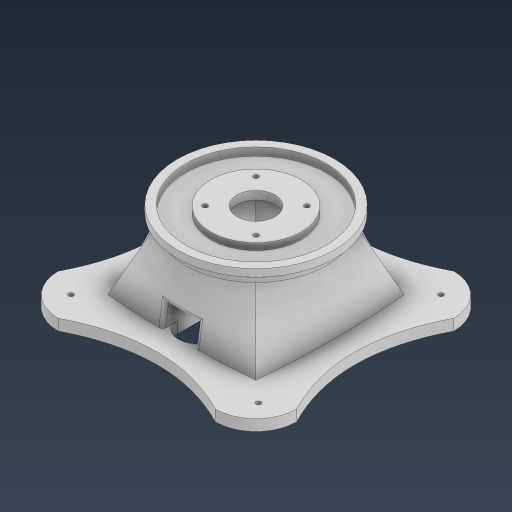
# Autodesk Inventor part: base_support
Saved by Autodesk Inventor 2024 (Build 280153000, 153)
## iProperties
Created: 2025-01-17
Part Number: base_support
Material: Generic
Document SubType Name: Modeling
Designer: Piter
Density: 1 g/cm^3
Appearance: Default
Author: Piter
Autodesk Inventor part; units mm, degrees
ref_plane "YZ Plane" through (0, 0, 0) normal (1, 0, 0) x (0, 1, 0)
sketch "Sketch1" plane through (0, 0, 0) normal (0, 1, 0) x (-1, 0, 0)
  circle A0 centre (0, 0) radius 27.35
  dimension "d0" = 54.7
  constraints: 1 centre point, 1 coincident
  measures "d0" diameter of A0
extrude "Extrusion1" add sketch "Sketch1" along normal blind 5
sketch "Sketch2" plane through (0, 0, 0) normal (0, -1, 0) x (1, 0, 0)
  circle A0 centre (0, 0) radius 47.5
  circle A1 centre (0, 0) radius 42.6
  circle A2 centre (0, 0) radius 27.35 projected
  dimension "d3" = 95
  dimension "d4" = 85.2
  constraints: 2 centre point, 2 coincident
  measures "d3" diameter of A0
  measures "d4" diameter of A1
extrude "Extrusion2" add sketch "Sketch2" along normal blind 5 and the other way blind 1 contours A1
extrude "Extrusion3" add sketch "Sketch2" along normal blind 2 and the other way blind 5.75 contours A0
chamfer "Chamfer1" distance 4.5 distance2 3.25 1 edges at (-47.5, -2, 0) measured on face at (-2.3305, -2, 44.0051)
ref_plane "Work Plane1" through (0, -48.5, 0) normal (0, -1, 0) x (1, 0, 0)
sketch "Sketch3" plane through (0, -48.5, 0) normal (0, -1, 0) x (1, 0, 0)
  line L0 (-47.5, 47.5) -> (47.5, 47.5)
  line L1 (47.5, 47.5) -> (47.5, -47.5)
  line L2 (47.5, -47.5) -> (-47.5, -47.5)
  line L3 (-47.5, -47.5) -> (-47.5, 47.5)
  line L4 (-47.5, 47.5) -> (47.5, -47.5) construction
  line L5 (47.5, 47.5) -> (-47.5, -47.5) construction
  line L6 (-22.5, 22.5) -> (22.5, 22.5)
  line L7 (22.5, 22.5) -> (22.5, -22.5)
  line L8 (22.5, -22.5) -> (-22.5, -22.5)
  line L9 (-22.5, -22.5) -> (-22.5, 22.5)
  circle A0 centre (0, 0) radius 27.35 projected
  line L10 (-22.5, 22.5) -> (22.5, -22.5) construction
  line L11 (22.5, 22.5) -> (-22.5, -22.5) construction
  dimension "d15" = 95
  dimension "d16" = 95
  dimension "d17" = 45
  dimension "d18" = 45
  constraints: 24 end point, 4 midpoint, 4 parallel, 2 horizontal, 2 perpendicular
  measures "d15" distance of L1.end L2.end
  measures "d16" distance of L0.end L1.end
  measures "d17" distance of L7.end L8.end
  measures "d18" distance of L6.end L7.end
sketch "Sketch4" plane through (0, -5, 0) normal (0, -1, 0) x (1, 0, 0)
  circle A0 centre (0, 0) radius 42.6 projected
  circle A1 centre (0, 0) radius 27.35 projected
sketch "Sketch5" plane through (0, -48.5, 0) normal (0, -1, 0) x (1, 0, 0)
  line L0 (-47.5, 47.5) -> (47.5, 47.5)
  line L1 (47.5, 47.5) -> (47.5, -47.5)
  line L2 (47.5, -47.5) -> (-47.5, -47.5)
  line L3 (-47.5, -47.5) -> (-47.5, 47.5)
  line L4 (-47.5, 47.5) -> (47.5, -47.5) construction
  line L5 (47.5, 47.5) -> (-47.5, -47.5) construction
  point P0 (0, 0)
  dimension "d21" = 95
  dimension "d22" = 95
  constraints: 12 end point, 2 midpoint, 2 parallel, 1 horizontal, 1 perpendicular
  measures "d21" distance of L1.end L2.end
  measures "d22" distance of L0.end L1.end
loft "Loft1" add profiles "Sketch5" section 2 edges at (-42.6, -5, 0)
extrude "Extrusion5" cut sketch "Sketch3" against normal blind 48.5 contours L6 A0 L9 | L6 A0 L7 L8 L9 | L6 L7 A0 | A0 L8 L9 | L7 L8 A0
ref_plane "Work Plane2" through (0, 2.25, 0) normal (0, 1, 0) x (1, 0, 0)
sketch "Sketch6" plane through (0, -5, 0) normal (0, 1, 0) x (1, 0, 0)
  line L0 (-15.549, 22.5) -> (15.549, 22.5) projected
  arc A0 (15.549, 22.5) -> (-15.549, 22.5) centre (0, 0) ccw projected
  line L1 (-22.5, -15.549) -> (-22.5, 15.549) projected
  arc A1 (-22.5, 15.549) -> (-22.5, -15.549) centre (0, 0) ccw projected
  line L2 (22.5, 15.549) -> (22.5, -15.549) projected
  arc A2 (22.5, -15.549) -> (22.5, 15.549) centre (0, 0) ccw projected
  line L3 (15.549, -22.5) -> (-15.549, -22.5) projected
  arc A3 (-15.549, -22.5) -> (15.549, -22.5) centre (0, 0) ccw projected
extrude "Extrusion6" add sketch "Sketch6" along normal blind 5
sketch "Sketch7" plane through (-47.5, -48.5, 47.5) normal (0, -1, 0) x (1, 0, 0)
  line L0 (0, 0) -> (95, 0) projected
  line L1 (95, 0) -> (77.6227, -17.3773) projected
  circle A0 centre (95, 0) radius 24.5751
  line L2 (95, -95) -> (0, -95) projected
  circle A1 centre (95, -95) radius 24.5751
  circle A2 centre (47.5, -47.5) radius 42.6 projected
  line L3 (0, -95) -> (17.3773, -77.6227) projected
  circle A3 centre (0, -95) radius 24.5751
  line L4 (0, 0) -> (17.3773, -17.3773) projected
  circle A4 centre (0, 0) radius 24.5751
  line L5 (95, 24.5751) -> (47.5, 0) construction
  line L6 (47.5, 0) -> (0, 24.5751) construction
  spline S0 degree 2 poles (95, 24.5751) (47.5, 0) (0, 24.5751) knots 1 1 1 2 2 2
  circle A5 centre (47.5, -47.5) radius 47.5 projected
  line L7 (-24.5751, 0) -> (0, -47.5) construction
  line L8 (0, -47.5) -> (-24.5751, -95) construction
  spline S1 degree 2 poles (-24.5751, 0) (0, -47.5) (-24.5751, -95) knots 1 1 1 2 2 2
  line L9 (0, -119.5751) -> (47.5, -95) construction
  line L10 (47.5, -95) -> (95, -119.5751) construction
  spline S2 degree 2 poles (0, -119.5751) (47.5, -95) (95, -119.5751) knots 1 1 1 2 2 2
  line L11 (119.5751, 0) -> (95, -47.5) construction
  line L12 (95, -47.5) -> (119.5751, -95) construction
  spline S3 degree 2 poles (119.5751, 0) (95, -47.5) (119.5751, -95) knots 1 1 1 2 2 2
  circle A6 centre (-8.3793, 8.3793) radius 1.5
  circle A7 centre (-8.3793, -103.3793) radius 1.5
  circle A8 centre (103.3793, -103.3793) radius 1.5
  circle A9 centre (104.8793, 8.3793) radius 1.5
  dimension "d47" = 3
  dimension "d48" = 3
  dimension "d49" = 3
  dimension "d50" = 3
  constraints: 14 point on circle, 8 centre point, 2 midpoint, 2 point on line, 1 coincident, 1 tangent, 12 other
  measures "d47" diameter of A6
  measures "d48" diameter of A7
  measures "d49" diameter of A8
  measures "d50" diameter of A9
extrude "Extrusion7" add sketch "Sketch7" against normal blind 7 contours L4 A5 A4 S1 S0 L0 | L0 A4 A5 L4 | A4 S0 A0 L0 | L0 A5 A4 | A5 A4 L4 | L4 A4 A5 | L0 A0 A5 | A5 A0 A2 A4 | A2 A3 A5 A4 | A5 A3 S1 A4 | A0 S0 S3 A5 L1 L0 | L0 L1 A5 A0 | A5 L1 A0 | L1 A5 A0 | A0 A5 A1 A2 | A3 A5 L3 | A2 A1 A5 A3 | L3 A5 A3 | A5 L3 L2 A3 S2 S1 | A0 S3 A1 A5 | A1 A5 | A5 A3 L2 L3 | A5 L2 A3 | A1 S3 S2 A5 | A1 L2 A5 | L2 A1 S2 A3
sketch "Sketch8" plane through (0, 5, 0) normal (0, 1, 0) x (1, 0, 0)
  circle A0 centre (0, 0) radius 11.5
  circle A1 centre (0, 0) radius 21.75
  line L0 (15.3796, -15.3796) -> (-15.3796, -15.3796)
  line L1 (-15.3796, -15.3796) -> (-15.3796, 15.3796)
  line L2 (-15.3796, 15.3796) -> (15.3796, 15.3796)
  line L3 (15.3796, 15.3796) -> (15.3796, -15.3796)
  line L4 (15.3796, -15.3796) -> (-15.3796, 15.3796) construction
  line L5 (-15.3796, -15.3796) -> (15.3796, 15.3796) construction
  circle A2 centre (-15.3796, 15.3796) radius 1.55
  circle A3 centre (15.3796, 15.3796) radius 1.55
  circle A4 centre (15.3796, -15.3796) radius 1.55
  circle A5 centre (-15.3796, -15.3796) radius 1.55
  dimension "d37" = 43.5
  dimension "d36" = 23
  dimension "d38" = 3.1
  dimension "d39" = 3.1
  dimension "d40" = 3.1
  dimension "d41" = 3.1
  constraints: 12 end point, 6 coincident, 5 centre point, 2 midpoint, 2 parallel, 2 perpendicular, 1 horizontal, 3 other
  measures "d36" diameter of A0
  measures "d38" diameter of A2
  measures "d39" diameter of A3
  measures "d40" diameter of A4
  measures "d41" diameter of A5
extrude "Extrusion8" cut sketch "Sketch8" against normal blind 10 contours A0 | A3 L3 A1 | A1 A3 | A4 A1 | A1 L3 A4 | L2 A3 A1 | L3 A3 L2 | A1 A4 L0 | L0 A4 L3 | A2 L2 A1 | A1 A2 | A2 L1 L2 | A5 A1 | A1 L0 A5 | L0 L1 A5 | L1 A2 A1 | A1 A5 L1
move faces "Move1" translate (0, 0.3, 0) faces at (-34.9452, -48.5, -0.9897)
sketch "Sketch9" plane through (22.5, 0, 22.5) normal (0, 0, -1) x (-1, 0, 0)
  point P0 (22.5, 0)
sketch "Sketch10" plane through (22.5, 0, 22.5) normal (0, 0, -1) x (-1, 0, 0)
  line L0 (0, -48.2) -> (0, 0) projected
  line L1 (0, -48.2) -> (45, -48.2)
  line L2 (22.5, -48.2) -> (22.5, -28.2)
  line L3 (12.5, -28.2) -> (32.5, -28.2)
  line L4 (32.5, -28.2) -> (32.5, -48.2)
  line L5 (32.5, -48.2) -> (12.5, -48.2)
  line L6 (12.5, -48.2) -> (12.5, -28.2)
  line L7 (12.5, -28.2) -> (32.5, -48.2) construction
  line L8 (32.5, -28.2) -> (12.5, -48.2) construction
  point P0 (22.5, 0)
  point P1 (22.5, -38.2)
  dimension "d51" = 20
  dimension "d52" = 20
  constraints: 16 end point, 4 midpoint, 2 parallel, 1 horizontal, 1 perpendicular, 1 point on line, 1 vertical
  measures "d51" distance of L2.start L2.end
  measures "d52" distance of L4.end L5.end
extrude "Extrusion9" cut sketch "Sketch10" against normal blind 24.25
fillet "Fillet1" radius 2 3 edges at (10, -34.8335, 45.7382) (0.0001, -28.2, 45.2133) (-10, -34.8335, 45.7382)
fillet "Fillet2" radius 9.25 2 edges at (10, -44.85, 46.75) (-10, -44.85, 46.75)
body "Solid1"
